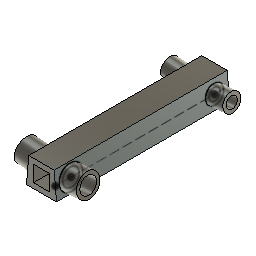
Wing to mainrod connector v2 (Autodesk Fusion 360 design; units mm, degrees)
Autodesk Fusion 360 part; units mm, degrees
sketch "Sketch1" plane through (0, 0, 0) normal (0, 1, 0) x (1, 0, 0)
  line L0 (3.8558, -6.289) -> (-5.3705, -6.289)
  line L1 (-5.3705, -6.289) -> (-5.3705, 2.9372)
  line L2 (-5.3705, 2.9372) -> (3.8558, 2.9372)
  line L3 (3.8558, 2.9372) -> (3.8558, -6.289)
  line L4 (6.5933, -9.289) -> (-8.1081, -9.289)
  line L5 (-8.1081, -9.289) -> (-9.4402, 5.9372)
  line L6 (-9.4402, 5.9372) -> (7.9254, 5.9372)
  line L7 (7.9254, 5.9372) -> (6.5933, -9.289)
  line L8 (-8.1081, -9.289) -> (6.5933, -9.289)
  line L9 (-5.3705, -6.289) -> (-8.3705, -6.289) construction
  line L10 (3.8558, -6.289) -> (6.8558, -6.289) construction
  dimension "d13" = 85
  dimension "d14" = 85
  dimension "d20" = 3
  dimension "d22" = 3
  dimension "d25" = 3
  dimension "d26" = 9.2263
  constraint equal L1 L2
  constraint horizontal L8
  constraint horizontal L0
  constraint equal L0 L1
  constraint coincident L5 L9.end
  constraint vertical L1
  constraint horizontal L9
  constraint vertical L3
  constraint equal L0 L3
  constraint coincident L7 L10.end
  constraint parallel L0 L10
  constraint equal L9 L10
  measures "d13" angle of L5 L6
  measures "d14" angle of L6 L7
  measures "d20" distance of L0.end L9.end
  measures "d22" distance of L0 L4
  measures "d25" distance of L2 L6
  measures "d26" distance of L0.start L2.end
extrude "Extrude1" add sketch "Sketch1" along normal blind 100
sketch "Sketch2" plane through (7.3497, 0, 0.643) normal (0.996195, 0, 0.087156) x (0, 1, 0)
  line L0 (0, 8.679) -> (0, -6.6054)
  line L1 (0, -6.6054) -> (100, -6.6054)
  line L2 (100, -6.6054) -> (100, 8.679)
  line L3 (100, 8.679) -> (0, 8.679)
  circle A0 centre (9, 1.0368) radius 4.775
  circle A1 centre (92.0226, 1.0368) radius 3.19
  line L4 (9, 1.0368) -> (0, 1.0368) construction
  line L5 (9, 1.0368) -> (92.0226, 1.0368) construction
  line L6 (92.0226, 1.0368) -> (100, 1.0368) construction
  circle A2 centre (9, 1.0368) radius 6.775
  circle A3 centre (92.0226, 1.0368) radius 5.19
  dimension "d29" = 83.0226
  dimension "d31" = 9.55
  dimension "d32" = 6.38
  dimension "d35" = 13.55
  dimension "d36" = 10.38
  dimension "d44" = 9
  constraint midpoint L0 L4.end
  constraint coincident A0.centre L4.start
  constraint coincident A1.centre L5.end
  constraint parallel L4 L5
  constraint midpoint L2 L6.end
  constraint perpendicular L2 L6
  constraint parallel L5 L6
  constraint concentric A0 A2
  constraint concentric A1 A3
  measures "d29" distance of A0.centre A1.centre
  measures "d31" diameter of A0
  measures "d32" diameter of A1
  measures "d35" diameter of A2
  measures "d36" diameter of A3
  measures "d44" distance of L0 A0.centre
extrude "Extrude2" add sketch "Sketch2" along normal blind 10 contours A2 | A3
sketch "Sketch3" plane through (-8.853, 0, 0.7745) normal (-0.996195, 0, 0.087156) x (0, -1, 0)
  line L0 (0, -6.7374) -> (0, 8.547)
  line L1 (0, 8.547) -> (-100, 8.547)
  line L2 (-100, 8.547) -> (-100, -6.7374)
  line L3 (-100, -6.7374) -> (0, -6.7374)
  circle A0 centre (-92.0226, 1.0368) radius 5.19
  circle A1 centre (-92.0226, 1.0368) radius 3.19
  circle A2 centre (-9, 1.0368) radius 4.775
  circle A3 centre (-9, 1.0368) radius 6.775
  dimension "d40" = 9.55
  dimension "d41" = 6.38
  dimension "d42" = 13.55
  dimension "d43" = 10.38
  dimension "d46" = 83.0226
  dimension "d47" = 9
  constraint concentric A2 A3
  constraint concentric A0 A1
  measures "d40" diameter of A2
  measures "d41" diameter of A1
  measures "d42" diameter of A3
  measures "d43" diameter of A0
  measures "d46" distance of A2.centre A0.centre
  measures "d47" distance of L0 A2.centre
extrude "Extrude3" add sketch "Sketch3" along normal blind 10 contours A0 | A3
equation "d35 = 9.55 mm + 4 mm"
equation "d36 = 6.38 mm + 4 mm"
equation "d42 = 9.55 mm + 4 mm"
equation "d43 = 6.38 mm + 4 mm"
